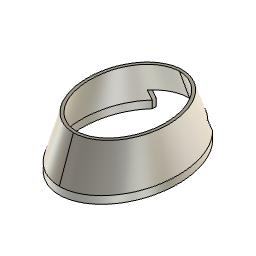
toothbrush_charger_case_v2 (Autodesk Fusion 360 design; units mm, degrees)
Autodesk Fusion 360 part; units mm, degrees
sketch "Sketch1" plane through (0, 0, 0) normal (0, 0, 1) x (1, 0, 0)
  line L0 (-10, 10) -> (-60, 10)
  line L1 (-60, 10) -> (-35, 10)
  line L2 (-35, 10) -> (-15, 10)
  line L3 (-15, 10) -> (-15, 37.5)
  line L4 (-15, 10) -> (-35, 10)
  line L5 (-35, 10) -> (-35, 37.5)
  line L6 (-35, 37.5) -> (-15, 37.5)
  line L7 (-15, 37.5) -> (-15, 10)
  ellipse E0 centre (-35, 37.5) end of major axis (-35, 10) minor radius 20
  line L8 (-35, 65) -> (-35, 10) construction
  line L9 (-55, 37.5) -> (-15, 37.5) construction
  line L10 (-10, 10) -> (-60, 10)
  line L11 (-60, 10) -> (-60, 72.5)
  line L12 (-60, 72.5) -> (-10, 72.5)
  line L13 (-10, 72.5) -> (-10, 10)
  line L14 (-10, 10) -> (-60, 10)
  line L15 (-60, 2.5) -> (-10, 2.5)
  line L16 (-10, 2.5) -> (-60, 2.5)
  line L17 (-10, 10) -> (-60, 10)
  line L18 (-60, 10) -> (-60, 2.5)
  line L19 (-60, 2.5) -> (-10, 2.5)
  line L20 (-10, 2.5) -> (-10, 10)
  ellipse E1 centre (-35, 37.5) end of major axis (-35, 2.5) minor radius 25
  line L21 (-35, 72.5) -> (-35, 2.5) construction
  line L22 (-60, 37.5) -> (-10, 37.5) construction
  ellipse E2 centre (-35, 37.5) end of major axis (-35, 74) minor radius 26.5
  line L23 (-35, 1) -> (-35, 74) construction
  line L24 (-8.5, 37.5) -> (-61.5, 37.5) construction
  dimension "d6" = 20
  dimension "d7" = 27.5
  dimension "d8" = 27.5
  dimension "d12" = 50
  dimension "d13" = 62.5
  dimension "d20" = 50
  dimension "d21" = 7.5
  dimension "d34" = 73
  dimension "d35" = 53
  constraint horizontal L0
  constraint parallel L0 L2
  constraint perpendicular L2 L3
  constraint horizontal L4
  constraint vertical L5
  constraint horizontal L6
  constraint vertical L7
  constraint coincident E0 L8.start
  constraint coincident E0 L1.end
  constraint coincident E0 L9.start
  constraint coincident E0 L3.end
  constraint coincident L5.end L6.start
  constraint coincident L1.end L2.start
  constraint perpendicular L0 L8
  constraint coincident L3.end L6.end
  constraint horizontal L10
  constraint vertical L11
  constraint horizontal L12
  constraint vertical L13
  constraint horizontal L14
  constraint horizontal L15
  constraint horizontal L16
  constraint horizontal L17
  constraint vertical L18
  constraint horizontal L19
  constraint vertical L20
  constraint coincident E1 L21.start
  constraint coincident E1 L21.end
  constraint coincident E1 L22.start
  constraint coincident E1 L22.end
  constraint concentric E0 E1
  constraint perpendicular L15 L21
  constraint coincident E2 L23.start
  constraint coincident E2 L23.end
  constraint coincident E2 L24.start
  constraint coincident E2 L24.end
  constraint concentric E1 E2
  constraint perpendicular L12 L23
  measures "d6" distance of L1.end L2.end
  measures "d7" distance of L2.end L3.end
  measures "d8" distance of L2.end L3.end
  measures "d12" distance of L0.start L0.end
  measures "d13" distance of L0.start L12.end
  measures "d20" distance of L0.start L0.end
  measures "d21" distance of L0.start L15.end
  measures "d34" distance of E2
extrude "Extrude4" add sketch "Sketch1" along normal blind 21 contours L5 L6 E0 | L5 L6 E0 makes body 1
sketch "Sketch4" plane through (0, 0, 21) normal (0, 0, 1) x (-1, 0, 0)
  ellipse E0 centre (35, -37.5) end of major axis (35, -10) minor radius 20
  ellipse E1 centre (35, -37.5) end of major axis (15, -37.5) minor radius 27.5
  line L0 (55, -37.5) -> (15, -37.5) construction
  line L1 (35, -10) -> (35, -65) construction
  ellipse E2 centre (35, -37.5) end of major axis (35, -66.5) minor radius 21.5
  line L2 (35, -8.5) -> (35, -66.5) construction
  line L3 (13.5, -37.5) -> (56.5, -37.5) construction
  dimension "d32" = 58
  dimension "d33" = 43
  constraint coincident E1 L0.start
  constraint coincident E1 L0.end
  constraint coincident E1 L1.start
  constraint coincident E1 L1.end
  constraint concentric E0 E1
  constraint horizontal L0
  constraint coincident E2 L2.start
  constraint coincident E2 L2.end
  constraint coincident E2 L3.start
  constraint coincident E2 L3.end
  constraint concentric E1 E2
  constraint perpendicular L0 L2
  measures "d32" distance of E2
extrude "Extrude5" cut 1 faces at (-28.4436, 39.7311, 0) along direction (0, 0, 1) blind 21 on bodies 1 bodies 1
loft "Loft2" add profiles "Sketch4", "Sketch1" section 1 section 2 contours L3 L7 L13 E1 E2 | L13 E2 | L0 L2 L4 L10 L14 L15 L16 L17 L19 E1 E2 | L0 L2 L3 L4 L7 L10 L14 L17 E1 E2 | L12 L13 E1 E2 | L15 L16 L19 E2 | L11 L12 E1 E2 | L12 E2 | L0 L1 L10 L14 L15 L16 L17 L19 E1 E2 | L0 L1 L10 L11 L14 L17 E1 E2 | L11 E2 separate body makes body 2
loft "Loft3" cut profiles "Sketch4", "Sketch1" section 1 contours E0 E1 section 2 contours L0 L1 L3 L7 E0 L10 L14 L17 E1 | L0 L1 L2 L4 L10 L14 L17 E1 | L0 L2 L3 L4 L7 E0 L10 L14 L17 E1 bodies 2
extrude "Extrude6" add 1 faces at (-59.1949, 26.6804, 0) along direction (0, 0, -1) blind 4 on bodies 2 bodies 1 2
sketch "Sketch5" plane through (0, 0, -4) normal (0, 0, -1) x (1, 0, 0)
  spline S0 degree 3 poles (-35, -72.5) (-38.5411, -72.5) (-42.0803, -71.4311) (-45.3064, -69.3874) (-48.6124, -67.293) (-51.5857, -64.1766) (-53.9521, -60.3255) (-55.5622, -57.7052) (-56.8928, -54.7489) (-57.8864, -51.5847) (-59.222, -47.3309) (-59.9442, -42.7017) (-59.9969, -38.0556) (-60.0677, -31.8097) (-58.9163, -25.545) (-56.701, -20.1226) (-55.4128, -16.9696) (-53.7714, -14.1) (-51.8552, -11.651) (-49.6535, -8.8372) (-47.0893, -6.5814) (-44.3233, -5.0249) (-41.1454, -3.2367) (-37.7028, -2.3763) (-34.2792, -2.5146) (-30.3457, -2.6734) (-26.4426, -4.156) (-22.9912, -6.8024) (-19.0257, -9.8429) (-15.669, -14.4211) (-13.3943, -19.8915) (-12.1623, -22.8545) (-11.2435, -26.0724) (-10.6773, -29.408) (-10.0714, -32.9778) (-9.8698, -36.6816) (-10.0824, -40.3387) (-10.3099, -44.2527) (-11.0122, -48.1117) (-12.1503, -51.7008) (-13.3682, -55.542) (-15.0853, -59.0717) (-17.1922, -62.0653) (-19.4471, -65.269) (-22.1476, -67.8557) (-25.0975, -69.6373) (-28.2138, -71.5193) (-31.6061, -72.5) (-35, -72.5) knots -1 -1 -1 -1 -0.93237 -0.93237 -0.93237 -0.863068 -0.863068 -0.863068 -0.815915 -0.815915 -0.815915 -0.752527 -0.752527 -0.752527 -0.66731 -0.66731 -0.66731 -0.617757 -0.617757 -0.617757 -0.560824 -0.560824 -0.560824 -0.495411 -0.495411 -0.495411 -0.420254 -0.420254 -0.420254 -0.333904 -0.333904 -0.333904 -0.287133 -0.287133 -0.287133 -0.237077 -0.237077 -0.237077 -0.183507 -0.183507 -0.183507 -0.126176 -0.126176 -0.126176 -0.064818 -0.064818 -0.064818 0 0 0 0
  ellipse E0 centre (-35, -37.5) end of major axis (-35, -74) minor radius 26.5
  line L0 (-35, -74) -> (-20, -74)
  line L1 (-20, -74) -> (-50, -74)
  line L2 (-50, -74) -> (-50, -59)
  line L3 (-50, -59) -> (-20, -59)
  line L4 (-20, -59) -> (-20, -74)
  dimension "d38" = 15
  dimension "d39" = 30
  dimension "d40" = 15
  constraint coincident E0 L0.start
  constraint horizontal L0
  constraint horizontal L1
  constraint vertical L2
  constraint horizontal L3
  constraint vertical L4
  measures "d38" distance of L0.start L0.end
  measures "d39" distance of L0.end L1.end
  measures "d40" distance of L0.end L3.end
extrude "Extrude7" cut sketch "Sketch5" against normal blind 10 contours S0 E0 L2 L4 | S0 L2 L3 L4 | E0 L1 L2 | E0 L0 L1 L4 picked at (-20.7424, -66.8909) picked at (-35, -63.5) bodies 1
